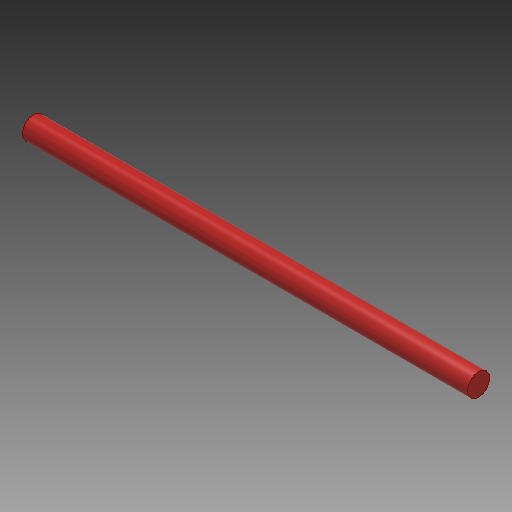
# Autodesk Inventor part: sim_shaft
Saved by Autodesk Inventor 2018.1 (Build 221171000, 171)
## iProperties
Created: 2017-10-27
Part Number: sim_shaft
Material: アルミニウム 6061
Document SubType Name: Modeling
Designer: Kakeru Yamashita
Density: 2.7 g/cm^3
Appearance: オレンジ-赤
Mass: 42.4115 g
Surface Area: 64.4026 cm^2
Volume: 15.708 cm^3
Author: Kakeru Yamashita
Autodesk Inventor part; units mm, degrees
ref_plane "YZ Plane" through (0, 0, 0) normal (1, 0, 0) x (0, 1, 0)
ref_plane "XZ Plane" through (0, 0, 0) normal (0, 1, 0) x (-1, 0, 0)
ref_plane "XY Plane" through (0, 0, 0) normal (0, 0, 1) x (1, 0, 0)
sketch "スケッチ1" plane through (0, 0, 0) normal (0, 1, 0) x (-1, 0, 0)
  point P0 (0, 0)
sketch "スケッチ2" plane through (0, 0, 0) normal (0, 1, 0) x (-1, 0, 0)
  circle A0 centre (0, 0) radius 5
  dimension "d0" = 10
  constraints: 1 centre point, 1 coincident
  measures "d0" diameter of A0
extrude "押し出し1" add sketch "スケッチ2" along normal blind 200
